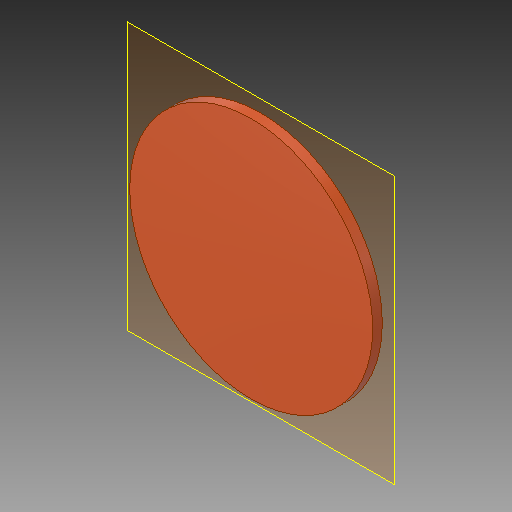
# Autodesk Inventor part: trapdoor
Saved by Autodesk Inventor 2019 (Build 230136000, 136)
## iProperties
Created: 2019-01-08
Part Number: trapdoor
Material: PET Plastic
Document SubType Name: Modeling
Designer: jmc
Density: 1.541 g/cm^3
Appearance: Smooth - Light Orange
Author: jmc
Autodesk Inventor part; units mm, degrees
ref_plane "YZ Plane" through (0, 0, 0) normal (1, 0, 0) x (0, 1, 0)
ref_plane "XZ Plane" through (0, 0, 0) normal (0, 1, 0) x (-1, 0, 0)
ref_plane "XY Plane" through (0, 0, 0) normal (0, 0, 1) x (1, 0, 0)
ref_plane "Work Plane1" through (0, 0, 0) normal (0, 0, 1) x (1, 0, 0)
sketch "Sketch1" plane through (0, 0, 0) normal (0, 0, 1) x (1, 0, 0)
  circle A0 centre (25.15, 0) radius 25.15 construction
  circle A1 centre (25.15, 0) radius 25.15 construction
  circle A2 centre (25.15, 0) radius 25.15
  point P0 (0, 0)
  constraints: 2 centre point, 2 coincident, 1 concentric, 1 horizontal alignment, 1 other
extrude "Extrusion1" add sketch "Sketch1" along normal blind 2
body "Solid1"
